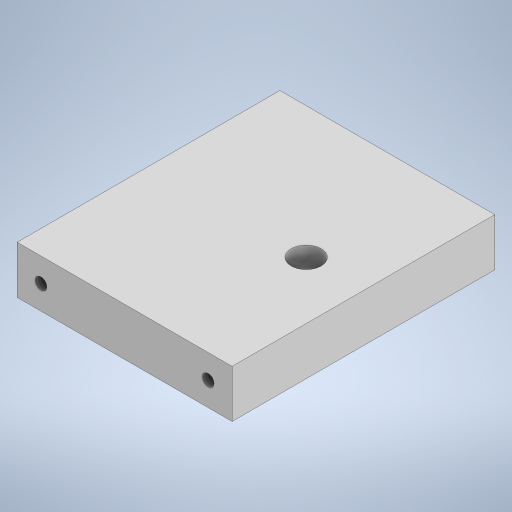
# Autodesk Inventor part: camera_connect_part
Saved by Autodesk Inventor 2024.3 (Build 283343010, 343A)
## iProperties
Created: 2025-07-19
Part Number: camera_connect_part
Material: 一般
Document SubType Name: Modeling
Designer: hikou
Density: 1 g/cm^3
Appearance: 既定
Author: hikou
Autodesk Inventor part; units mm, degrees
ref_plane "YZ Plane" through (0, 0, 0) normal (1, 0, 0) x (0, 1, 0)
ref_plane "XZ Plane" through (0, 0, 0) normal (0, 1, 0) x (-1, 0, 0)
ref_plane "XY Plane" through (0, 0, 0) normal (0, 0, 1) x (1, 0, 0)
sketch "スケッチ1" plane through (0, 0, 0) normal (0, 0, 1) x (1, 0, 0)
  line L0 (-22.5, -5) -> (22.5, -5)
  line L1 (22.5, -5) -> (22.5, 5)
  line L2 (22.5, 5) -> (-22.5, 5)
  line L3 (-22.5, 5) -> (-22.5, -5)
  line L4 (-22.5, -5) -> (22.5, 5) construction
  line L5 (22.5, -5) -> (-22.5, 5) construction
  point P0 (0, 0)
  dimension "d0" = 45
  dimension "d1" = 10
  constraints: 12 end point, 2 midpoint, 2 parallel, 1 horizontal, 1 perpendicular
  measures "d0" distance of L2.end L1.end
  measures "d1" distance of L1.end L0.end
extrude "押し出し1" add sketch "スケッチ1" along normal mid plane 55
sketch "スケッチ2" plane through (0, 0, 27.5) normal (0, 0, 1) x (1, 0, 0)
  line L0 (22.5, 5) -> (-22.5, 5) projected
  line L1 (-22.5, 5) -> (-22.5, -5) projected
  line L2 (22.5, -5) -> (22.5, 5) projected
  point P0 (0, 0)
  point P1 (-17.5, 0)
  point P2 (17.5, 0)
  dimension "d4" = 5
  dimension "d5" = 5
  dimension "d6" = 5
  dimension "d7" = 5
  measures "d4" distance from line of L0 point (-17.5, 0)
  measures "d5" distance from line of L1 point (-17.5, 0)
  measures "d6" distance from line of L2 point (17.5, 0)
  measures "d7" distance from line of L0 point (17.5, 0)
hole "穴1" at (-17.5, 0, 27.5) at (17.5, 0, 27.5) direction (0, 0, -1) diameter 2.459 depth 8.8 tip angle 118 thread size "M3x0.5" class "6H" standard "ISO Metric profile"
sketch "スケッチ3" plane through (0, 0, -27.5) normal (0, 0, -1) x (-1, 0, 0)
  line L0 (-22.5, 5) -> (-22.5, -5) projected
  line L1 (-22.5, -5) -> (22.5, -5) projected
  line L2 (22.5, -5) -> (22.5, 5) projected
  line L3 (22.5, 5) -> (-22.5, 5) projected
  circle A0 centre (-17.5, 0) radius 1.2295 projected
  circle A1 centre (17.5, 0) radius 1.2295 projected
  point P0 (0, 0)
  constraints: 2 coincident
hole "穴2" at (17.5, 0, -27.5) at (-17.5, 0, -27.5) direction (0, 0, 1) diameter 2.459 depth 8.8 tip angle 118 thread size "M3x0.5" class "6H" standard "ISO Metric profile"
sketch "スケッチ4" plane through (-22.5, 5, 27.5) normal (0, 1, 0) x (1, 0, 0)
  line L0 (45, 55) -> (45, 0) projected
  line L1 (45, 0) -> (0, 0) projected
  point P0 (22.5, 27.5)
  point P1 (33, 27.5)
  dimension "d22" = 12
  dimension "d23" = 27.5
  measures "d22" distance from line of L0 point (33, 27.5)
  measures "d23" distance from line of L1 point (33, 27.5)
hole "穴3" at (10.5, 5, 0) direction (0, -1, 0) diameter 6.3 end through all
equation "\"d5\" = d4"
equation "\"d6\" = d4"
equation "\"d7\" = d4"
